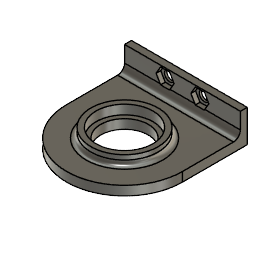
Anterior da Solenoide (Autodesk Fusion 360 design; units mm, degrees)
Autodesk Fusion 360 part; units mm, degrees
sketch "Esboço1" plane through (0, 0, 0) normal (0, 0, 1) x (1, 0, 0)
  line L0 (25, 28) -> (-25, 28)
  line L1 (-25, 0) -> (-25, 28)
  line L2 (25, 0) -> (25, 28)
  arc A0 (-25, 0) -> (25, 0) centre (0, 0) ccw
  circle A1 centre (0, 0) radius 10.25
  dimension "d1" = 50
  dimension "d3" = 28
  dimension "d4" = 20.5
  constraint coincident A0.centre A1.centre
  constraint horizontal L0
  constraint tangent L1 A0
  constraint tangent L2 A0
  constraint vertical L2
  constraint equal L1 L2
  measures "d1" diameter of A0
  measures "d3" distance of L0.end L1.start
  measures "d4" diameter of A1
extrude "Extrusão1" add sketch "Esboço1" along normal blind 4
sketch "Esboço2" plane through (0, 0, 4) normal (0, 0, 1) x (-1, 0, 0)
  circle A0 centre (0, 0) radius 10.25
  arc A1 (25, 0) -> (-25, 0) centre (0, 0) ccw
  line L0 (-25, 0) -> (-25, -28)
  line L1 (-25, -28) -> (25, -28)
  line L2 (25, -28) -> (25, 0)
  line L3 (25, -28) -> (-25, -28)
  line L4 (-25, -28) -> (-25, -25)
  line L5 (-25, -25) -> (25, -25)
  line L6 (25, -25) -> (25, -28)
  dimension "d7" = 3
  constraint horizontal L3
  constraint vertical L4
  constraint horizontal L5
  constraint vertical L6
  constraint coincident L0 L4.end
  constraint coincident L1.end L2.start
  measures "d7" distance of L1.end L5.end
extrude "Extrusão2" add sketch "Esboço2" along normal blind 10 contours L0 L1 L2 L3 L4 L5 L6
fillet "Arredondamento2" radius 3 1 edges at (0, 25, 4)
sketch "Esboço3" plane through (0, 28, 0) normal (0, 1, 0) x (-1, 0, 0)
  line L0 (-25, 0) -> (25, 0)
  line L1 (25, 0) -> (25, 14)
  line L2 (25, 14) -> (-25, 14)
  line L3 (-25, 14) -> (-25, 0)
  circle A0 centre (-7.5, 10) radius 2.25
  line L4 (0, -15) -> (0, 41) construction
  circle A1 centre (7.5, 10) radius 2.25
  dimension "d14" = 4.5
  dimension "d15" = 10
  dimension "d25" = 7.5
  constraint perpendicular L0 L4
  constraint symmetric A0 L4 A1
  constraint coincident origin L4
  measures "d14" diameter of A0
  measures "d15" distance of L0 A0.centre
  measures "d25" distance of A0.centre L4
extrude "Extrusão3" cut sketch "Esboço3" against normal up to surface (3 mm away) contours A0 | A1
sketch "Esboço4" plane through (0, 0, 4) normal (0, 0, 1) x (-1, 0, 0)
  line L0 (-25, -22) -> (25, -22)
  line L1 (25, -22) -> (25, 0)
  arc A0 (25, 0) -> (-25, 0) centre (0, 0) ccw
  line L2 (-25, 0) -> (-25, -22)
  circle A1 centre (0, 0) radius 10.25
  circle A2 centre (0, 0) radius 12.25
  circle A3 centre (0, 0) radius 14.5
  dimension "d19" = 24.5
  dimension "d20" = 29
  constraint concentric A0 A2
  constraint concentric A2 A3
  measures "d19" diameter of A2
  measures "d20" diameter of A3
extrude "Extrusão4" add sketch "Esboço4" along normal blind 4 contours A3
fillet "Arredondamento3" radius 2 1 edges at (13.5187, -5.2434, 4)
sketch "Esboço5" plane through (0, 25, 0) normal (0, -1, 0) x (1, 0, 0)
  circle A0 centre (7.5, 10) radius 2.25
  circle A1 centre (-7.5, 10) radius 2.25
  line L0 (-25, 7) -> (25, 7)
  line L1 (25, 7) -> (25, 14)
  line L2 (25, 14) -> (-25, 14)
  line L3 (-25, 14) -> (-25, 7)
  line L4 (-5.566, 13.3498) -> (-9.434, 13.3498)
  line L5 (-9.434, 13.3498) -> (-11.368, 10)
  line L6 (-11.368, 10) -> (-9.434, 6.6502)
  line L7 (-9.434, 6.6502) -> (-5.566, 6.6502)
  line L8 (-5.566, 6.6502) -> (-3.632, 10)
  line L9 (-3.632, 10) -> (-5.566, 13.3498)
  line L10 (0, 0) -> (0, 14) construction
  line L11 (3.632, 10) -> (5.566, 13.3498)
  line L12 (5.566, 13.3498) -> (9.434, 13.3498)
  line L13 (9.434, 13.3498) -> (11.368, 10)
  line L14 (11.368, 10) -> (9.434, 6.6502)
  line L15 (9.434, 6.6502) -> (5.566, 6.6502)
  line L16 (5.566, 6.6502) -> (3.632, 10)
  point P0 (-7.5, 10)
  dimension "d26" = 7.736
  constraint coincident P0 A1.centre
  constraint horizontal L4
  constraint coincident L10.start origin
  constraint midpoint L2 L10.end
  constraint symmetric L4.start L10 L11.end
  constraint symmetric L4.end L10 L12.end
  constraint symmetric L5.end L10 L13.end
  constraint symmetric L6.end L10 L14.end
  constraint symmetric L7.end L10 L15.end
  constraint symmetric L8.end L10 L11.start
  measures "d26" distance of L4.start L6.end
extrude "Extrusão5" cut sketch "Esboço5" along normal mid plane 4 contours L0 L4 L5 L6 L8 L9 | L0 L6 L7 L8 | L0 L11 L12 L13 L14 L16 | L0 L14 L15 L16
equation "d8 = 7.75 mm + ( 4.5 / 2 ) * 1 mm"
equation "d15 = 7.75 mm + ( 4.5 / 2 ) * 1 mm"
equation "d25 = ( 15 / 2 ) * 1 mm"
